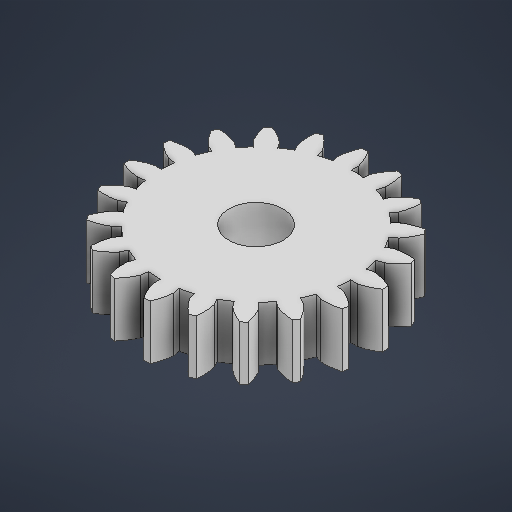
# Autodesk Inventor part: 40mm_20N_Gear
Saved by Autodesk Inventor 2026.2 (Build 302298000, 298)
## iProperties
Created: 2025-12-17
Part Number: 40mm_20N_Gear
Material: Generic
Document SubType Name: Modeling
Designer: Cobble
Density: 1 g/cm^3
Appearance: Default
Author: Cobble
Autodesk Inventor part; units mm, degrees
ref_plane "YZ Plane" through (0, 0, 0) normal (1, 0, 0) x (0, 1, 0)
ref_plane "XZ Plane" through (0, 0, 0) normal (0, 1, 0) x (-1, 0, 0)
ref_plane "XY Plane" through (0, 0, 0) normal (0, 0, 1) x (1, 0, 0)
sketch "Sketch1" plane through (0, 0, 0) normal (0, 0, 1) x (1, 0, 0)
  line L0 (0, 0) -> (0, 20) construction
  line L1 (0, 0) -> (20, 0) construction
  line L2 (0, 0) -> (20, 0) construction
  line L3 (0, 0) -> (-6.1803, 19.0211) construction
  line L4 (0, 0) -> (-11.7557, 16.1803) construction
  line L5 (0, 0) -> (-16.1803, 11.7557) construction
  line L6 (0, 0) -> (-19.0211, 6.1803) construction
  line L7 (0, 0) -> (-20, 0) construction
  line L8 (0, 0) -> (-19.0211, -6.1803) construction
  line L9 (0, 0) -> (-16.1803, -11.7557) construction
  line L10 (0, 0) -> (-11.7557, -16.1803) construction
  line L11 (0, 0) -> (-6.1803, -19.0211) construction
  line L12 (0, 0) -> (0, -20) construction
  line L13 (0, 0) -> (6.1803, -19.0211) construction
  line L14 (0, 0) -> (11.7557, -16.1803) construction
  line L15 (0, 0) -> (16.1803, -11.7557) construction
  line L16 (0, 0) -> (19.0211, -6.1803) construction
  line L17 (0, 0) -> (20, 0) construction
  line L18 (0, 0) -> (19.0211, 6.1803) construction
  line L19 (0, 0) -> (16.1803, 11.7557) construction
  line L20 (0, 0) -> (11.7557, 16.1803) construction
  line L21 (0, 0) -> (6.1803, 19.0211) construction
  line L22 (0, 0) -> (22, 0) construction
  line L23 (0, 0) -> (22, 0) construction
  circle A0 centre (0, 0) radius 17
  circle A1 centre (0, 0) radius 17.5
  circle A2 centre (0, 0) radius 22
  line L24 (-5.8075, 17.8737) -> (-0.1925, 19.6981) construction
  line L25 (-11.0465, 15.2043) -> (-1.4937, 22.1448) construction
  line L26 (-15.2043, 11.0465) -> (-4.7934, 25.3759) construction
  line L27 (-17.8737, 5.8075) -> (-10.5759, 28.2677) construction
  line L28 (-18.7935, 0) -> (-18.7935, 29.52) construction
  line L29 (-17.8737, -5.8075) -> (-28.8203, 27.8827) construction
  spline S0 degree 4 poles (0, 18.7935) (0.022, 19.368) (-0.8979, 22.081) (-5.8921, 27.4195) (-15.4945, 30.4627) (-23.1398, 29.6505) (-28.8203, 27.8827) knots 0 0 0 0 0 0.292815 0.46534 1 1 1 1 1 construction
  line L30 (0, 0) -> (-3.1287, 19.7538) construction
  line L31 (0, 0) -> (20, 0) construction
  arc A3 (-5.5118, 19.2255) -> (0, 20) centre (0, 0) ccw construction
  arc A4 (-5.5118, 19.2255) -> (0, 20) centre (0, 0) ccw construction
  arc A5 (0, 16.9334) -> (0.009, 17) centre (-6.5932, 17.8635) ccw
  line L32 (0, 18.7935) -> (0, 0) construction
  line L33 (-1.3628, 21.9578) -> (-1.274, 19.9594) construction
  line L34 (-0.7658, 20.9831) -> (-1.3201, 20.9978) construction
  arc A6 (-1.963, 22.7393) -> (0.3545, 17.4964) centre (-9.6703, 16.1989) ccw construction
  arc A7 (-0.3029, 19.9977) -> (-3.1287, 19.7538) centre (0, 0) ccw construction
  arc A8 (-5.5118, 19.2255) -> (0, 20) centre (0, 0) ccw construction
  line L35 (0, 19.1425) -> (0, 18.7935)
  line L36 (0, 0) -> (22, 0) construction
  arc A9 (-4.962, 25.1438) -> (0.3545, 17.4964) centre (-9.6703, 16.1989) ccw construction
  arc A10 (0.0995, 18.7932) -> (-1.3628, 21.9578) centre (-9.6703, 16.1989) ccw
  line L37 (-1.7201, 19.9259) -> (0, 0) construction
  arc A11 (-2.4204, 21.8665) -> (-3.3187, 18.4982) centre (6.7511, 17.6165) ccw
  line L38 (-3.3187, 18.4982) -> (0, 0)
  line L39 (0.0995, 18.7932) -> (0, 0)
  arc A12 (-5.7128, 17.9042) -> (-8.0814, 20.4619) centre (-14.2027, 12.4178) ccw
  arc A13 (-9.059, 20.0483) -> (-8.8725, 16.5673) centre (0.9769, 18.8405) ccw
  line L40 (-8.8725, 16.5673) -> (0, 0)
  line L41 (-5.7128, 17.9042) -> (0, 0)
  arc A14 (-10.9659, 15.2625) -> (-14.009, 16.9632) centre (-17.3449, 7.4212) ccw
  arc A15 (-14.8109, 16.2677) -> (-13.5578, 13.0146) centre (-4.893, 18.2202) ccw
  line L42 (-13.5578, 13.0146) -> (0, 0)
  line L43 (-10.9659, 15.2625) -> (0, 0)
  arc A16 (-15.1456, 11.1269) -> (-18.5652, 11.8039) centre (-18.7892, 1.6981) ccw
  arc A17 (-19.113, 10.8947) -> (-16.916, 8.1881) centre (-10.2838, 15.8165) ccw
  line L44 (-16.916, 8.1881) -> (0, 0)
  line L45 (-15.1456, 11.1269) -> (0, 0)
  arc A18 (-17.8427, 5.902) -> (-21.3042, 5.4892) centre (-18.3943, -4.1912) ccw
  arc A19 (-21.5442, 4.4552) -> (-18.6183, 2.56) centre (-14.6681, 11.8645) ccw
  line L46 (-18.6183, 2.56) -> (0, 0)
  line L47 (-17.8427, 5.902) -> (0, 0)
  arc A20 (-18.7932, 0.0995) -> (-21.9578, -1.3628) centre (-16.1989, -9.6703) ccw
  arc A21 (-21.8665, -2.4204) -> (-18.4982, -3.3187) centre (-17.6165, 6.7511) ccw
  line L48 (-18.4982, -3.3187) -> (0, 0)
  line L49 (-18.7932, 0.0995) -> (0, 0)
  arc A22 (-17.9042, -5.7128) -> (-20.4619, -8.0814) centre (-12.4178, -14.2027) ccw
  arc A23 (-20.0483, -9.059) -> (-16.5673, -8.8725) centre (-18.8405, 0.9769) ccw
  line L50 (-16.5673, -8.8725) -> (0, 0)
  line L51 (-17.9042, -5.7128) -> (0, 0)
  arc A24 (-15.2625, -10.9659) -> (-16.9632, -14.009) centre (-7.4212, -17.3449) ccw
  arc A25 (-16.2677, -14.8109) -> (-13.0146, -13.5578) centre (-18.2202, -4.893) ccw
  line L52 (-13.0146, -13.5578) -> (0, 0)
  line L53 (-15.2625, -10.9659) -> (0, 0)
  arc A26 (-11.1269, -15.1456) -> (-11.8039, -18.5652) centre (-1.6981, -18.7892) ccw
  arc A27 (-10.8947, -19.113) -> (-8.1881, -16.916) centre (-15.8165, -10.2838) ccw
  line L54 (-8.1881, -16.916) -> (0, 0)
  line L55 (-11.1269, -15.1456) -> (0, 0)
  arc A28 (-5.902, -17.8427) -> (-5.4892, -21.3042) centre (4.1912, -18.3943) ccw
  arc A29 (-4.4552, -21.5442) -> (-2.56, -18.6183) centre (-11.8645, -14.6681) ccw
  line L56 (-2.56, -18.6183) -> (0, 0)
  line L57 (-5.902, -17.8427) -> (0, 0)
  arc A30 (-0.0995, -18.7932) -> (1.3628, -21.9578) centre (9.6703, -16.1989) ccw
  arc A31 (2.4204, -21.8665) -> (3.3187, -18.4982) centre (-6.7511, -17.6165) ccw
  line L58 (3.3187, -18.4982) -> (0, 0)
  line L59 (-0.0995, -18.7932) -> (0, 0)
  arc A32 (5.7128, -17.9042) -> (8.0814, -20.4619) centre (14.2027, -12.4178) ccw
  arc A33 (9.059, -20.0483) -> (8.8725, -16.5673) centre (-0.9769, -18.8405) ccw
  line L60 (8.8725, -16.5673) -> (0, 0)
  line L61 (5.7128, -17.9042) -> (0, 0)
  arc A34 (10.9659, -15.2625) -> (14.009, -16.9632) centre (17.3449, -7.4212) ccw
  arc A35 (14.8109, -16.2677) -> (13.5578, -13.0146) centre (4.893, -18.2202) ccw
  line L62 (13.5578, -13.0146) -> (0, 0)
  line L63 (10.9659, -15.2625) -> (0, 0)
  arc A36 (15.1456, -11.1269) -> (18.5652, -11.8039) centre (18.7892, -1.6981) ccw
  arc A37 (19.113, -10.8947) -> (16.916, -8.1881) centre (10.2838, -15.8165) ccw
  line L64 (16.916, -8.1881) -> (0, 0)
  line L65 (15.1456, -11.1269) -> (0, 0)
  arc A38 (17.8427, -5.902) -> (21.3042, -5.4892) centre (18.3943, 4.1912) ccw
  arc A39 (21.5442, -4.4552) -> (18.6183, -2.56) centre (14.6681, -11.8645) ccw
  line L66 (18.6183, -2.56) -> (0, 0)
  line L67 (17.8427, -5.902) -> (0, 0)
  arc A40 (18.7932, -0.0995) -> (21.9578, 1.3628) centre (16.1989, 9.6703) ccw
  arc A41 (21.8665, 2.4204) -> (18.4982, 3.3187) centre (17.6165, -6.7511) ccw
  line L68 (18.4982, 3.3187) -> (0, 0)
  line L69 (18.7932, -0.0995) -> (0, 0)
  arc A42 (17.9042, 5.7128) -> (20.4619, 8.0814) centre (12.4178, 14.2027) ccw
  arc A43 (20.0483, 9.059) -> (16.5673, 8.8725) centre (18.8405, -0.9769) ccw
  line L70 (16.5673, 8.8725) -> (0, 0)
  line L71 (17.9042, 5.7128) -> (0, 0)
  arc A44 (15.2625, 10.9659) -> (16.9632, 14.009) centre (7.4212, 17.3449) ccw
  arc A45 (16.2677, 14.8109) -> (13.0146, 13.5578) centre (18.2202, 4.893) ccw
  line L72 (13.0146, 13.5578) -> (0, 0)
  line L73 (15.2625, 10.9659) -> (0, 0)
  arc A46 (11.1269, 15.1456) -> (11.8039, 18.5652) centre (1.6981, 18.7892) ccw
  arc A47 (10.8947, 19.113) -> (8.1881, 16.916) centre (15.8165, 10.2838) ccw
  line L74 (8.1881, 16.916) -> (0, 0)
  line L75 (11.1269, 15.1456) -> (0, 0)
  arc A48 (5.902, 17.8427) -> (5.4892, 21.3042) centre (-4.1912, 18.3943) ccw
  arc A49 (4.4552, 21.5442) -> (2.56, 18.6183) centre (11.8645, 14.6681) ccw
  line L76 (2.56, 18.6183) -> (0, 0)
  line L77 (5.902, 17.8427) -> (0, 0)
  point P0 (-1.3432, 21.959)
  point P1 (-2.4399, 21.8643)
  point P2 (5.4078, -16.6435)
  point P3 (5.8075, -17.8737)
  point P4 (0, -17.5)
  point P5 (0, -18.7935)
  point P6 (-5.4078, -16.6435)
  point P7 (-5.8075, -17.8737)
  point P8 (-10.2862, -14.1578)
  point P9 (-11.0465, -15.2043)
  point P10 (-14.1578, -10.2862)
  point P11 (-15.2043, -11.0465)
  point P12 (-16.6435, -5.4078)
  point P13 (-17.5, 0)
  point P14 (-16.6435, 5.4078)
  point P15 (-14.1578, 10.2862)
  point P16 (-10.2862, 14.1578)
  point P17 (-5.4078, 16.6435)
  point P18 (0, 17.5)
  point P19 (-2.94, 18.5621)
  point P20 (-2.7376, 17.2845)
  point P21 (5.4078, 16.6435)
  point P22 (5.8075, 17.8737)
  point P23 (10.2862, 14.1578)
  point P24 (11.0465, 15.2043)
  point P25 (10.2862, -14.1578)
  point P26 (11.0465, -15.2043)
  point P27 (14.1578, -10.2862)
  point P28 (15.2043, -11.0465)
  point P29 (16.6435, -5.4078)
  point P30 (17.8737, -5.8075)
  point P31 (14.1578, 10.2862)
  point P32 (15.2043, 11.0465)
  point P33 (16.6435, 5.4078)
  point P34 (17.8737, 5.8075)
  point P35 (17.5, 0)
  point P36 (18.7935, 0)
  point P37 (17.5, 0)
  point P38 (-18.6815, 11.619)
  point P39 (-15.5693, 7.9904)
  point P40 (-3.0903, 17.225)
  point P41 (-5.3196, 16.6719)
  point P42 (-8.0814, 20.4619)
  point P43 (-9.059, 20.0483)
  point P44 (-8.2618, 15.427)
  point P45 (-10.2112, 14.212)
  point P46 (-14.009, 16.9632)
  point P47 (-14.8109, 16.2677)
  point P48 (-12.6247, 12.1189)
  point P49 (-14.1031, 10.361)
  point P50 (-18.5652, 11.8039)
  point P51 (-19.113, 10.8947)
  point P52 (-15.7517, 7.6245)
  point P53 (-16.6146, 5.4958)
  point P54 (-21.3042, 5.4892)
  point P55 (-21.5442, 4.4552)
  point P56 (-17.3369, 2.3838)
  point P57 (-17.4998, 0.0926)
  point P58 (-21.9578, -1.3628)
  point P59 (-21.8665, -2.4204)
  point P60 (-17.225, -3.0903)
  point P61 (-16.6719, -5.3196)
  point P62 (-20.4619, -8.0814)
  point P63 (-20.0483, -9.059)
  point P64 (-15.427, -8.2618)
  point P65 (-14.212, -10.2112)
  point P66 (-16.9632, -14.009)
  point P67 (-16.2677, -14.8109)
  point P68 (-12.1189, -12.6247)
  point P69 (-10.361, -14.1031)
  point P70 (-11.8039, -18.5652)
  point P71 (-10.8947, -19.113)
  point P72 (-7.6245, -15.7517)
  point P73 (-5.4958, -16.6146)
  point P74 (-5.4892, -21.3042)
  point P75 (-4.4552, -21.5442)
  point P76 (-2.3838, -17.3369)
  point P77 (-0.0926, -17.4998)
  point P78 (1.3628, -21.9578)
  point P79 (2.4204, -21.8665)
  point P80 (3.0903, -17.225)
  point P81 (5.3196, -16.6719)
  point P82 (8.0814, -20.4619)
  point P83 (9.059, -20.0483)
  point P84 (8.2618, -15.427)
  point P85 (10.2112, -14.212)
  point P86 (14.009, -16.9632)
  point P87 (14.8109, -16.2677)
  point P88 (12.6247, -12.1189)
  point P89 (14.1031, -10.361)
  point P90 (18.5652, -11.8039)
  point P91 (19.113, -10.8947)
  point P92 (15.7517, -7.6245)
  point P93 (16.6146, -5.4958)
  point P94 (21.3042, -5.4892)
  point P95 (21.5442, -4.4552)
  point P96 (17.3369, -2.3838)
  point P97 (17.4998, -0.0926)
  point P98 (21.9578, 1.3628)
  point P99 (21.8665, 2.4204)
  point P100 (17.225, 3.0903)
  point P101 (16.6719, 5.3196)
  point P102 (20.4619, 8.0814)
  point P103 (20.0483, 9.059)
  point P104 (15.427, 8.2618)
  point P105 (14.212, 10.2112)
  point P106 (16.9632, 14.009)
  point P107 (16.2677, 14.8109)
  point P108 (12.1189, 12.6247)
  point P109 (5.4958, 16.6146)
  point P110 (5.4892, 21.3042)
  point P111 (4.4552, 21.5442)
  point P112 (2.3838, 17.3369)
  point P113 (0.0926, 17.4998)
  point P114 (-2.4204, 21.8665)
  point P115 (10.361, 14.1031)
  point P116 (11.8039, 18.5652)
  point P117 (10.8947, 19.113)
  point P118 (7.6245, 15.7517)
  dimension "d29" = 34
  dimension "d30" = 35
  dimension "d32" = 44
  dimension "d34" = 37.587
  dimension "d35" = 5.904
  dimension "d36" = 11.808
  dimension "d37" = 17.712
  dimension "d38" = 23.616
  dimension "d41" = 29.52
  dimension "d42" = 35.424
  dimension "d43" = 99
  dimension "d53" = 20
  dimension "d66" = 360
  constraints: 156 end point, 96 point on circle, 47 centre point, 14 point on line, 8 coincident, 6 horizontal, 6 perpendicular, 3 symmetric about line, 2 collinear, 2 vertical, 1 equal length, 322 other
  measures "d35" distance of L24.start L24.end
  measures "d36" distance of L25.end L25.start
  measures "d37" distance of L26.start L26.end
  measures "d38" distance of L27.start L27.end
  measures "d41" distance of L28.start L28.end
  measures "d42" distance of L29.start L29.end
  measures "d43" angle of L31 L30
  measures "d53" radius of A4
extrude "Extrusion1" add sketch "Sketch1" along normal blind 10 contours A0 L69 L68 | A0 L68 A1 L69 | L68 L71 A0 | A0 L71 A1 L68 | L69 A1 L66 A0 | A0 L66 L69 | L71 L70 A0 | A0 L70 A1 L71 | L68 A41 A2 A40 L69 A1 | L41 A0 L38 | L38 A0 L39 | L43 A0 L40 | L40 A0 L41 | L45 A0 L42 | L42 A0 L43 | L47 A0 L44 | L44 A0 L45 | L49 A0 L46 | L46 A0 L47 | L51 A0 L48 | L48 A0 L49 | L53 A0 L50 | L50 A0 L51 | L55 A0 L52 | L52 A0 L53 | L57 A0 L54 | L54 A0 L55 | L59 A0 L56 | L56 A0 L57 | L61 A0 L58 | L58 A0 L59 | L63 A0 L60 | L60 A0 L61 | L65 A0 L62 | L62 A0 L63 | L67 A0 L64 | L64 A0 L65 | L66 A0 L67 | L73 A0 L70 | L75 A0 L72 | L72 A0 L73 | L77 A0 L74 | L74 A0 L75 | L39 A0 L76 | L76 A0 L77 | L66 A1 L67 A0 | A0 L73 A1 L70 | A1 L70 A43 A2 A42 L71 | L38 A1 L39 A0 | A0 L41 A1 L38 | L39 A1 L76 A0 | L40 A1 L41 A0 | A0 L43 A1 L40 | L42 A1 L43 A0 | A0 L45 A1 L42 | L44 A1 L45 A0 | A0 L47 A1 L44 | L46 A1 L47 A0 | A0 L49 A1 L46 | L48 A1 L49 A0 | A0 L51 A1 L48 | L50 A1 L51 A0 | A0 L53 A1 L50 | L52 A1 L53 A0 | A0 L55 A1 L52 | L54 A1 L55 A0 | A0 L57 A1 L54 | L56 A1 L57 A0 | A0 L59 A1 L56 | L58 A1 L59 A0 | A0 L61 A1 L58 | L60 A1 L61 A0 | A0 L63 A1 L60 | L62 A1 L63 A0 | A0 L65 A1 L62 | L64 A1 L65 A0 | A0 L67 A1 L64 | L72 A1 L73 A0 | A0 L75 A1 L72 | L74 A1 L75 A0 | A0 L77 A1 L74 | L76 A1 L77 A0 | L66 A39 A2 A38 L67 A1 | L38 A11 A2 A10 L39 A1 | L40 A13 A2 A12 L41 A1 | L42 A15 A2 A14 L43 A1 | L44 A17 A2 A16 L45 A1 | L46 A19 A2 A18 L47 A1 | L48 A21 A2 A20 L49 A1 | L50 A23 A2 A22 L51 A1 | L52 A25 A2 A24 L53 A1 | L54 A27 A2 A26 L55 A1 | L56 A29 A2 A28 L57 A1 | L58 A31 A2 A30 L59 A1 | L60 A33 A2 A32 L61 A1 | L62 A35 A2 A34 L63 A1 | L64 A37 A2 A36 L65 A1 | L72 A45 A2 A44 L73 A1 | L74 A47 A2 A46 L75 A1 | L76 A49 A2 A48 L77 A1
sketch "Sketch2" plane through (0, 0, 10) normal (0, 0, 1) x (1, 0, 0)
  circle A0 centre (0, 0) radius 5
  dimension "d50" = 10
  constraints: 1 centre point, 1 coincident
  measures "d50" diameter of A0
extrude "Extrusion2" cut sketch "Sketch2" against normal blind 10
body "Solid1"
